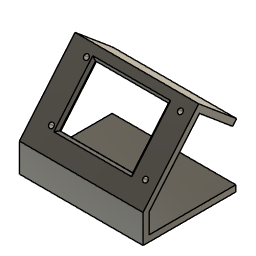
pico-arduino-env-mon_case (Autodesk Fusion 360 design; units mm, degrees)
Autodesk Fusion 360 part; units mm, degrees
sketch "スケッチ2" plane through (0, 0, 0) normal (1, 0, 0) x (0, 1, 0)
  line L0 (0, 0) -> (75, 0)
  line L1 (75, 0) -> (75, 5)
  line L2 (0, 0) -> (0, 23.1027)
  line L3 (0, 23.1027) -> (44.9951, 76.7258)
  line L4 (44.9951, 76.7258) -> (48.8254, 73.5119)
  line L5 (45.6114, 69.6816) -> (12.2109, 29.8764)
  line L6 (75, 5) -> (5, 5)
  line L7 (5, 5) -> (5, 21.2828)
  line L8 (12.2109, 29.8764) -> (5, 21.2828)
  line L9 (48.8254, 73.5119) -> (75.6369, 51.0143)
  line L10 (75.6369, 51.0143) -> (72.423, 47.1841)
  line L11 (72.423, 47.1841) -> (45.6114, 69.6816)
  line L12 (72.423, 47.1841) -> (38.998, 7.3498)
  line L13 (38.998, 7.3498) -> (12.1865, 29.8473)
  dimension "d1" = 140
  dimension "d7" = 5
  dimension "d8" = 70
  dimension "d9" = 5
  dimension "d11" = 52
  dimension "d12" = 70
  dimension "d57" = 5
  dimension "d73" = 35
  constraint coincident L0.start L2.start
  constraint horizontal L0
  constraint perpendicular L0 L1
  constraint perpendicular L1 L6
  constraint perpendicular L0 L2
  constraint perpendicular L4 L5
  constraint horizontal L6
  constraint perpendicular L6 L7
  constraint parallel L5 L8
  constraint perpendicular L3 L4
  constraint perpendicular L5 L11
  constraint perpendicular L9 L10
  constraint perpendicular L10 L11
  constraint coincident L5 L13.end
  constraint perpendicular L5 L13
  constraint perpendicular L12 L13
  measures "d1" angle of L2 L3
  measures "d7" distance of L9.end L10.end
  measures "d8" distance of L2.end L3.end
  measures "d9" distance of L2 L7
  measures "d11" distance of L10.end L12.end
  measures "d12" distance of L1.end L6.end
  measures "d57" distance of L3 L5
  measures "d73" distance of L10 L5.start
extrude "押し出し1" add sketch "スケッチ2" along normal blind 100 contours L0 L1 L2 L3 L4 L5 L6 L7 L8 L9 L10 L11
sketch "スケッチ3" plane through (0, -11.3759, 9.5455) normal (0, -0.766044, 0.642788) x (1, 0, 0)
  line L0 (0, 87.6977) -> (0, 17.6977)
  line L1 (0, 17.6977) -> (100, 17.6977)
  line L2 (100, 17.6977) -> (100, 87.6977)
  line L3 (100, 87.6977) -> (0, 87.6977)
  line L4 (18, 81.6977) -> (87, 81.6977)
  line L5 (87, 81.6977) -> (87, 31.6977)
  line L6 (87, 31.6977) -> (18, 31.6977)
  line L7 (18, 31.6977) -> (18, 81.6977)
  line L8 (20.5, 79.1977) -> (79.5, 79.1977)
  line L9 (79.5, 79.1977) -> (79.5, 34.1977)
  line L10 (79.5, 34.1977) -> (20.5, 34.1977)
  line L11 (20.5, 34.1977) -> (20.5, 79.1977)
  line L12 (15, 78.6977) -> (91, 78.6977)
  line L13 (91, 78.6977) -> (91, 34.6977)
  line L14 (91, 34.6977) -> (15, 34.6977)
  line L15 (15, 34.6977) -> (15, 78.6977)
  circle A0 centre (15, 34.6977) radius 3
  circle A1 centre (15, 78.6977) radius 3
  circle A2 centre (91, 78.6977) radius 3
  circle A3 centre (91, 34.6977) radius 3
  dimension "d15" = 69
  dimension "d16" = 50
  dimension "d17" = 59
  dimension "d18" = 45
  dimension "d19" = 2.5
  dimension "d20" = 2.5
  dimension "d29" = 44
  dimension "d30" = 3
  dimension "d31" = 76
  dimension "d33" = 3
  dimension "d34" = 6
  dimension "d35" = 20.5
  dimension "d69" = 6
  constraint horizontal L4
  constraint vertical L5
  constraint horizontal L6
  constraint vertical L7
  constraint horizontal L8
  constraint vertical L9
  constraint horizontal L10
  constraint vertical L11
  constraint parallel L3 L12
  constraint perpendicular L3 L13
  constraint perpendicular L13 L14
  constraint perpendicular L12 L15
  constraint coincident L14.end L15.start
  constraint tangent L7 A0
  constraint coincident L12.start L15.end
  constraint tangent L7 A1
  constraint coincident L12.end L13.start
  constraint coincident L13.end L14.start
  measures "d15" distance of L4.start L4.end
  measures "d16" distance of L4.start L6.end
  measures "d17" distance of L8.start L8.end
  measures "d18" distance of L8.start L10.end
  measures "d19" distance of L7 L11
  measures "d20" distance of L6 L10
  measures "d29" vertical distance of L12.start L14.end
  measures "d30" distance of L6 L14
  measures "d31" distance of L12.start L12.end
  measures "d33" distance of L7 L15
  measures "d34" distance of L3 L4
  measures "d35" distance of L0 L11
  measures "d69" diameter of A2
extrude "押し出し2" cut sketch "スケッチ3" against normal blind 5 contours L9 L11 L12 L14 | L8 L9 L11 L12 | L9 L10 L11 L14
extrude "押し出し3" cut sketch "スケッチ3" along normal blind 2 from surface at -5 contours L4 L5 L7 L8 L9 L11 L12 | L7 L11 L12 L14 | L5 L9 L12 L14 | L5 L6 L7 L9 L10 L11 L14
move_face "面をオフセット1" offset -1 1 faces at (41, 44.4579, 69.3441)
extrude "押し出し5" add sketch "スケッチ3" against normal blind 2 from surface at -5 contours L12 L15 A1 | L12 L15 A1
move_face "面をオフセット2" offset -1 1 faces at (18, 32.8056, 56.4945)
move_face "面をオフセット3" offset -1 1 faces at (87, 34.1733, 57.0874)
move_face "面をオフセット4" offset -1 1 faces at (64.3333, 11.8079, 31.4704)
chamfer "面取り1" distance 2 angle 45 4 edges at (79.5, 25.0687, 52.9784) (50, 39.5314, 70.2144) (20.5, 25.0687, 52.9784) (50, 10.606, 35.7424)
move_face "面をオフセット5" offset -2 1 faces at (17.2778, 42.6339, 66.1331)
extrude "押し出し6" add sketch "スケッチ3" against normal blind 2 from surface at -5 contours L14 L15 A0 | L14 L15 A0
extrude "押し出し7" add sketch "スケッチ3" against normal blind 2 from surface at -5 contours L12 L13 A2 | L12 L13 A2 | L13 L14 A3 | L13 L14 A3
hole "穴1" at (15, 39.21, 69.8314) direction (0, 0.766044, -0.642788) diameter 4 depth 8 tip angle 118
hole "穴2" at (91, 39.21, 69.8314) direction (0, 0.766044, -0.642788) diameter 4 depth 7 tip angle 118
hole "穴3" at (91, 10.9274, 36.1254) direction (0, 0.766044, -0.642788) diameter 4 depth 7 tip angle 118
hole "穴4" at (15, 10.9274, 36.1254) direction (0, 0.766044, -0.642788) diameter 4 depth 7 tip angle 118
move_face "面をオフセット6" offset -2 1 faces at (17.6569, 14.8474, 33.0185)
equation "d35 = ( ( 100 - 59 ) / 2 ) * 1 mm"
named bodies: "body"
